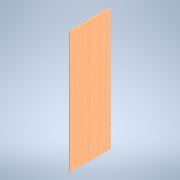
# Autodesk Inventor part: leftside
Saved by Autodesk Inventor 2020 (Build 240168000, 168)
## iProperties
Created: 2020-05-02
Part Number: leftside
Material: Generic
Document SubType Name: Modeling
Designer: galaxy
Density: 1 g/cm^3
Appearance: Default
Author: galaxy
Autodesk Inventor part; units mm, degrees
ref_plane "YZ Plane" through (0, 0, 0) normal (1, 0, 0) x (0, 1, 0)
ref_plane "XZ Plane" through (0, 0, 0) normal (0, 1, 0) x (-1, 0, 0)
ref_plane "XY Plane" through (0, 0, 0) normal (0, 0, 1) x (1, 0, 0)
sketch "Sketch1" plane through (0, 0, 0) normal (1, 0, 0) x (0, 1, 0)
  line L0 (180, 100) -> (-180, 100)
  line L1 (-180, 100) -> (-180, -100)
  line L2 (-180, -100) -> (180, -100)
  line L3 (180, -100) -> (180, 100)
  line L4 (180, 100) -> (-180, -100) construction
  line L5 (-180, 100) -> (180, -100) construction
  point P0 (0, 0)
  dimension "d0" = 360
  dimension "d1" = 200
  constraints: 12 end point, 2 midpoint, 2 parallel, 1 horizontal, 1 perpendicular
  measures "d0" distance of L2.end L1.end
  measures "d1" distance of L1.end L0.end
extrude "Extrusion1" add sketch "Sketch1" along normal blind 3
sketch "Sketch5" plane through (3, 0, 0) normal (1, 0, 0) x (0, 0, -1)
  circle A0 centre (0, 170) radius 1.875
  circle A1 centre (0, 144.2) radius 1.875
  circle A2 centre (0, 118.4) radius 1.875
  line L0 (100, 180) -> (-100, 180) projected
  line L1 (-100, 180) -> (-100, -180) projected
  line L2 (100, -180) -> (100, 180) projected
  circle A3 centre (0, -170) radius 1.875
  circle A4 centre (0, -144.2) radius 1.875
  circle A5 centre (0, -118.4) radius 1.875
  line L3 (-100, -180) -> (100, -180) projected
  line L4 (-100, -180) -> (100, -180)
  dimension "d46" = 10
  dimension "d47" = 25.8
  dimension "d48" = 25.8
  constraints: 6 centre point, 2 end point, 1 collinear
  measures "d46" distance from line of L0 A0.centre
  measures "d47" distance of A0.centre A1.centre
  measures "d48" distance of A1.centre A2.centre
extrude "Extrusion8" cut sketch "Sketch5" against normal blind 3 contours A0 | A1 | A2 | A3 | A4 | A5
sketch "Sketch6" plane through (3, 0, 0) normal (1, 0, 0) x (0, 0, -1)
  line L0 (100, 180) -> (-100, 180) projected
  line L1 (-100, 180) -> (-20, 180)
  line L2 (-20, 180) -> (-20, -170.3754)
  line L3 (-20, 180) -> (330.3754, 180) construction
  line L4 (-20, -170.3754) -> (-20, -180)
  line L5 (-100, -180) -> (100, -180) projected
  line L6 (-20, -180) -> (-100, -180)
  line L7 (-100, 180) -> (-100, -180) projected
  line L8 (-100, 180) -> (-100, -180)
  point P0 (0, 0)
  dimension "d65" = 80
  dimension "d66" = 90
  constraints: 12 end point, 3 point on line, 2 collinear, 1 horizontal, 1 perpendicular
  measures "d65" distance of L0.end L1.end
  measures "d66" angle of L2 L3
extrude "Extrusion9" cut sketch "Sketch6" against normal blind 3
body "Solid1"
